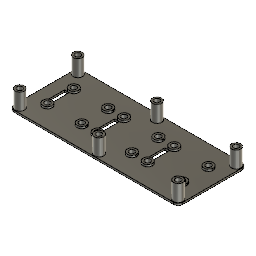
smmb_led-matrix-holder (Autodesk Fusion 360 design; units mm, degrees)
Autodesk Fusion 360 part; units mm, degrees
sketch "Sketch3" plane through (0, 0, 0) normal (0, 0, 1) x (1, 0, 0)
  line L0 (0, 0) -> (32, 0)
  line L1 (32, 0) -> (32, 32)
  line L2 (32, 32) -> (0, 32)
  line L3 (0, 32) -> (0, 0)
  line L4 (-0.5, 32.5) -> (-0.5, -0.5)
  line L5 (-0.5, -0.5) -> (32.5, -0.5)
  line L6 (32.5, -0.5) -> (32.5, 32.5)
  line L7 (32.5, 32.5) -> (-0.5, 32.5)
  line L8 (70, 32) -> (38, 32)
  line L9 (38, 32) -> (38, 0)
  line L10 (37.5, -0.5) -> (70.5, -0.5)
  line L11 (70.5, 32.5) -> (37.5, 32.5)
  line L12 (70, 0) -> (70, 32)
  line L13 (70.5, -0.5) -> (70.5, 32.5)
  line L14 (38, 0) -> (70, 0)
  line L15 (37.5, 32.5) -> (37.5, -0.5)
  line L16 (108, 32) -> (76, 32)
  line L17 (76, 32) -> (76, 0)
  line L18 (75.5, -0.5) -> (108.5, -0.5)
  line L19 (108.5, 32.5) -> (75.5, 32.5)
  line L20 (108, 0) -> (108, 32)
  line L21 (108.5, -0.5) -> (108.5, 32.5)
  line L22 (76, 0) -> (108, 0)
  line L23 (75.5, 32.5) -> (75.5, -0.5)
  line L24 (38, 32) -> (70, 0)
  line L25 (70, 32) -> (38, 0)
  line L26 (118, -10) -> (-10, -10)
  line L27 (-10, -10) -> (-10, 42)
  line L28 (-10, 42) -> (118, 42)
  line L29 (118, 42) -> (118, -10)
  line L30 (118, -10) -> (-10, 42) construction
  line L31 (-10, -10) -> (118, 42) construction
  circle A0 centre (3, 26) radius 2.05
  circle A1 centre (3, 26) radius 3.55
  circle A2 centre (29, 26) radius 3.55
  circle A3 centre (29, 26) radius 2.05
  circle A4 centre (29, 6) radius 2.05
  circle A5 centre (29, 6) radius 3.55
  circle A6 centre (3, 6) radius 2.05
  circle A7 centre (3, 6) radius 3.55
  circle A8 centre (67, 6) radius 2.05
  circle A9 centre (67, 6) radius 3.55
  circle A10 centre (41, 6) radius 2.05
  circle A11 centre (41, 6) radius 3.55
  circle A12 centre (67, 26) radius 2.05
  circle A13 centre (67, 26) radius 3.55
  circle A14 centre (41, 26) radius 2.05
  circle A15 centre (41, 26) radius 3.55
  circle A16 centre (105, 6) radius 2.05
  circle A17 centre (105, 6) radius 3.55
  circle A18 centre (79, 6) radius 2.05
  circle A19 centre (79, 6) radius 3.55
  circle A20 centre (105, 26) radius 2.05
  circle A21 centre (105, 26) radius 3.55
  circle A22 centre (79, 26) radius 2.05
  circle A23 centre (79, 26) radius 3.55
  line L32 (3, 22.45) -> (-0.5, 22.45)
  line L33 (-0.5, 22.45) -> (-0.5, 9.55)
  line L34 (-0.5, 9.55) -> (3, 9.55)
  line L35 (3, 9.55) -> (3, 22.45)
  line L36 (41, 22.45) -> (37.5, 22.45)
  line L37 (41, 9.55) -> (41, 22.45)
  line L38 (37.5, 9.55) -> (41, 9.55)
  line L39 (37.5, 22.45) -> (37.5, 9.55)
  line L40 (79, 22.45) -> (75.5, 22.45)
  line L41 (79, 9.55) -> (79, 22.45)
  line L42 (75.5, 9.55) -> (79, 9.55)
  line L43 (75.5, 22.45) -> (75.5, 9.55)
  circle A24 centre (-6, 38) radius 2.05
  circle A25 centre (-6, 38) radius 3.55
  circle A26 centre (54, 38) radius 2.05
  circle A27 centre (54, 38) radius 3.55
  circle A28 centre (114, 38) radius 2.05
  circle A29 centre (114, 38) radius 3.55
  circle A30 centre (-6, -6) radius 2.05
  circle A31 centre (-6, -6) radius 3.55
  circle A32 centre (54, -6) radius 2.05
  circle A33 centre (54, -6) radius 3.55
  circle A34 centre (114, -6) radius 2.05
  circle A35 centre (114, -6) radius 3.55
  point P0 (38, 0)
  point P1 (76, 0)
  point P2 (54, 16)
  dimension "d57" = 32
  dimension "d58" = 32
  dimension "d59" = 0.5
  dimension "d62" = 76
  dimension "d63" = 0
  dimension "d66" = 10
  dimension "d67" = 10
  dimension "d68" = 4.1
  dimension "d69" = 3
  dimension "d70" = 6
  dimension "d71" = 7.1
  dimension "d74" = 26
  dimension "d75" = 0
  dimension "d78" = 0
  dimension "d79" = -20
  dimension "d82" = 76
  dimension "d83" = 0
  dimension "d84" = 3.5
  dimension "d85" = 12.9
  dimension "d86" = 9.55
  dimension "d89" = 76
  dimension "d90" = 0
  dimension "d95" = 4
  dimension "d96" = 4
  dimension "d97" = 4.1
  dimension "d98" = 7.1
  dimension "d101" = 120
  dimension "d102" = 0
  dimension "d105" = 0
  dimension "d106" = -44
  constraint horizontal L0
  constraint vertical L1
  constraint horizontal L2
  constraint vertical L3
  constraint coincident L0.start L3.end
  constraint coincident P0 L9.end
  constraint perpendicular L26 L27
  constraint parallel L26 L28
  constraint parallel L27 L29
  constraint horizontal L26
  constraint coincident L30 P2
  constraint coincident L31 P2
  constraint midpoint L24 P2
  constraint concentric A0 A1
  constraint horizontal L32
  constraint vertical L33
  constraint horizontal L34
  constraint vertical L35
  constraint coincident A1 L32.start
  constraint concentric A24 A25
  measures "d57" distance of L0.start L2.end
  measures "d58" distance of L0.start L0.end
  measures "d66" distance of L2 L28
  measures "d67" distance of L3 L27
  measures "d68" diameter of A0
  measures "d69" distance of L3 A0.centre
  measures "d70" distance of L2 A0.centre
  measures "d71" diameter of A1
  measures "d84" distance of L32.start L32.end
  measures "d85" distance of L32.start L34.end
  measures "d86" distance of L2 L32
  measures "d95" distance of L27 A24.centre
  measures "d96" distance of L28 A24.centre
  measures "d97" diameter of A24
  measures "d98" diameter of A25
extrude "Extrude1" add sketch "Sketch3" along normal blind 1.5 contours L0 L1 L2 L3 A1 A2 A5 A7 L35 | L0 L1 L3 L4 L5 L6 A5 A7 | L3 L4 A7 | L3 A7 | L1 A5 | L1 L6 A5 | L3 L4 A7 L34 | L3 A7 L34 | L4 A7 | L1 L6 A2 A5 | L6 A5 | L1 A2 | L1 L6 A2 | L3 L4 A1 L32 | L3 A1 L32 | L3 A1 | L1 L2 L3 L4 L6 L7 A1 A2 | L6 A2 | L3 L4 A1 | L4 A1 | L8 L24 L25 A13 A15 | L8 L9 L11 L12 L13 L15 A13 A15 | L12 L25 A13 | L9 L24 A15 | L12 L13 A13 | L12 L25 A13 | L25 A13 | L9 L24 A15 | L9 L15 A15 | L24 A15 | L12 L13 A9 A13 | L12 L24 L25 A9 A13 | L13 A13 | L9 A15 L36 | L9 L15 A15 L36 | L15 A15 | L24 L25 A11 A15 L37 | L12 L13 A9 | L12 L24 A9 | L14 L24 L25 A9 A11 | L9 L10 L12 L13 L14 L15 A9 A11 | L12 L24 A9 | L13 A9 | L24 A9 | L25 A11 | L9 L25 A11 | L9 A11 L38 | L9 L15 A11 L38 | L9 L25 A11 | L9 L15 A11 | L15 A11 | L16 L17 L20 L22 A17 A19 A21 A23 L41 | L16 L17 L19 L20 L21 L23 A21 A23 | L20 L21 A21 | L20 A21 | L17 A23 | L17 L23 A23 | L20 L21 A17 A21 | L21 A21 | L17 A23 L40 | L17 L23 A23 L40 | L23 A23 | L20 L21 A17 | L20 A17 | L17 L18 L20 L21 L22 L23 A17 A19 | L21 A17 | L17 A19 L42 | L17 L23 A19 L42 | L17 A19 | L17 L23 A19 | L23 A19 | L26 L27 L28 L29 | A24 | A25 | A26 | A27 | A28 | A29 | A30 | A31 | A32 | A33 | A34 | A35
extrude "Extrude2" add sketch "Sketch3" along normal blind 3 contours L3 L4 A7 | L3 A7 | L1 A5 | L1 L6 A5 | L1 A2 | L1 L6 A2 | L3 A1 | L3 L4 A1 | L12 L13 A13 | L12 L25 A13 | L25 A13 | L9 L24 A15 | L9 L15 A15 | L24 A15 | L12 L13 A9 | L12 L24 A9 | L24 A9 | L25 A11 | L9 L25 A11 | L9 L15 A11 | L20 L21 A21 | L20 A21 | L17 A23 | L17 L23 A23 | L20 L21 A17 | L20 A17 | L17 A19 | L17 L23 A19 picked at (69.6833, 26) picked at (38.3167, 26) picked at (69.6833, 6) picked at (38.3167, 6)
extrude "Extrude3" add sketch "Sketch3" along normal blind 14 contours A25 | A27 | A29 | A31 | A33 | A35
fillet "Fillet1" radius 3.5 4 edges at (118, -10, 0.75) (-10, -10, 0.75) (118, 42, 0.75) (-10, 42, 0.75)
equation "d71 = d68 + 3 mm"
equation "d97 = d68"
equation "d98 = d97 + 3 mm"
equation "d111 = 3 mm + 12.5 mm - 1.5 mm"
